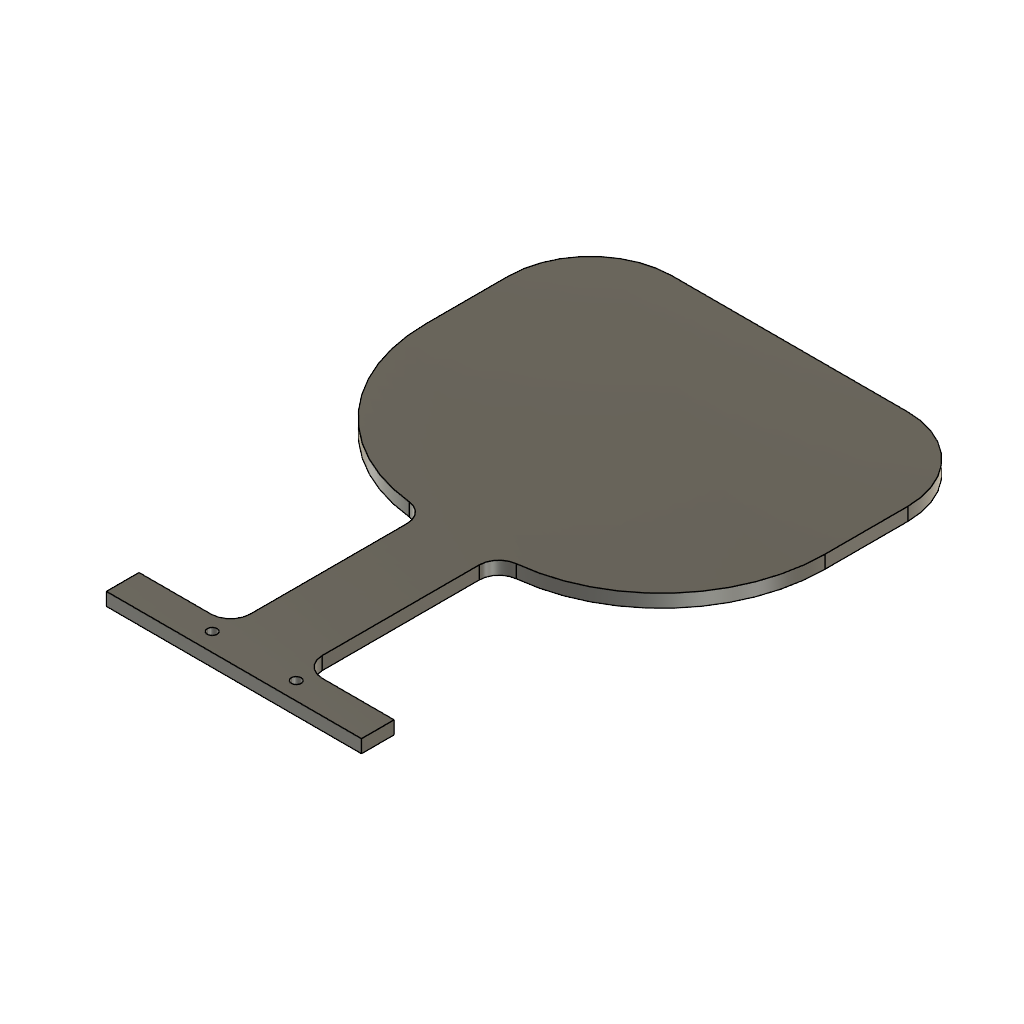
line follower robo chasis (Autodesk Fusion 360 design; units mm, degrees)
part number: 2026-06-19-20-18-20-474
Autodesk Fusion 360 part; units mm, degrees
sketch "Sketch1" plane through (0, 0, 0) normal (0, 0, 1) x (1, 0, 0)
  line L0 (-62, 100) -> (60, 100)
  line L1 (60, 100) -> (60, 0)
  line L2 (60, 0) -> (10, 0)
  line L3 (10, 0) -> (10, -60)
  line L4 (10, -60) -> (38, -60)
  line L5 (38, -60) -> (38, -70)
  line L6 (38, -70) -> (-40, -70)
  line L7 (-40, -70) -> (-40, -60)
  line L8 (-40, -60) -> (-12, -60)
  line L9 (-12, -60) -> (-12, 0)
  line L10 (-12, 0) -> (-62, 0)
  line L11 (-62, 0) -> (-62, 100)
  dimension "d1" = 28
  dimension "d2" = 28
  dimension "d3" = 78
  dimension "d4" = 50
  constraint horizontal L0
  constraint perpendicular L0 L1
  constraint perpendicular L1 L2
  constraint perpendicular L2 L3
  constraint perpendicular L1 L4
  constraint perpendicular L4 L5
  constraint perpendicular L3 L6
  constraint perpendicular L6 L7
  constraint perpendicular L3 L8
  constraint perpendicular L8 L9
  constraint perpendicular L9 L10
  constraint perpendicular L0 L11
  constraint equal L2 L10
  constraint equal L3 L9
  constraint equal L5 L7
  measures "d1" distance of L3.end L4.end
  measures "d2" distance of L7.end L8.end
  measures "d3" distance of L5.end L6.end
  measures "d4" distance of L9.end L10.end
extrude "Extrude1" add sketch "Sketch1" along normal blind 4
fillet "Fillet1" radius 25 2 edges at (60, 100, 2) (-62, 100, 2)
fillet "Fillet2" radius 6 4 edges at (10, 0, 2) (-12, 0, 2) (10, -60, 2) (-12, -60, 2)
hole "Hole1" at (-13.1996, -64.4309, 4) direction (0, 0, -1) diameter 3 depth 10 tip angle 180
hole "Hole2" at (12.6439, -64.5934, 4) direction (0, 0, -1) diameter 3 depth 10 tip angle 180
sketch "Sketch2" plane through (0, 0, 4) normal (0, 0, 1) x (-1, 0, 0)
  circle A0 centre (-12.6439, 64.5934) radius 1.5
  circle A1 centre (13.1996, 64.4309) radius 1.5
  arc A2 (37, -100) -> (62, -75) centre (37, -75) ccw
  line L0 (62, -75) -> (62, 0)
  line L1 (62, 0) -> (18, 0)
  arc A3 (12, 6) -> (18, 0) centre (18, 6) ccw
  line L2 (12, 6) -> (12, 54)
  arc A4 (18, 60) -> (12, 54) centre (18, 54) ccw
  line L3 (18, 60) -> (40, 60)
  line L4 (40, 60) -> (40, 70)
  line L5 (40, 70) -> (-38, 70)
  line L6 (-38, 70) -> (-38, 60)
  line L7 (-38, 60) -> (-16, 60)
  arc A5 (-10, 54) -> (-16, 60) centre (-16, 54) ccw
  line L8 (-10, 54) -> (-10, 6)
  arc A6 (-16, 0) -> (-10, 6) centre (-16, 6) ccw
  line L9 (-16, 0) -> (-60, 0)
  line L10 (-60, 0) -> (-60, -75)
  arc A7 (-60, -75) -> (-35, -100) centre (-35, -75) ccw
  line L11 (-35, -100) -> (37, -100)
  line L12 (62, -70) -> (57, -70)
  line L13 (57, -70) -> (57, -50)
  line L14 (57, -50) -> (62, -50)
  line L15 (62, -50) -> (62, -70)
  line L16 (32, -70) -> (32, -50)
  line L17 (37, -70) -> (32, -70)
  line L18 (37, -50) -> (37, -70)
  line L19 (32, -50) -> (37, -50)
  line L20 (-60, -70) -> (-60, -50)
  line L21 (-55, -70) -> (-60, -70)
  line L22 (-55, -50) -> (-55, -70)
  line L23 (-60, -50) -> (-55, -50)
  line L24 (-35, -70) -> (-35, -50)
  line L25 (-30, -70) -> (-35, -70)
  line L26 (-30, -50) -> (-30, -70)
  line L27 (-35, -50) -> (-30, -50)
  dimension "d17" = 5
  dimension "d18" = 20
  dimension "d19" = 30
  dimension "d20" = 5
  dimension "d21" = 20
  dimension "d22" = 30
  dimension "d23" = 5
  dimension "d24" = 20
  dimension "d25" = 5
  dimension "d26" = 20
  dimension "d27" = 25
  constraint horizontal L12
  constraint vertical L13
  constraint horizontal L14
  constraint vertical L15
  constraint coincident L0 L12.start
  constraint horizontal L17
  constraint vertical L16
  constraint horizontal L19
  constraint vertical L18
  constraint horizontal L25
  constraint vertical L24
  constraint horizontal L27
  constraint vertical L26
  constraint horizontal L21
  constraint vertical L20
  constraint horizontal L23
  constraint vertical L22
  measures "d17" distance of L12.start L12.end
  measures "d18" distance of L12.start L14.end
  measures "d19" distance of L11 L12
  measures "d20" distance of L17.start L16.start
  measures "d21" distance of L17.start L18.start
  measures "d22" distance of L0 L16
  measures "d23" distance of L25.start L24.start
  measures "d24" distance of L25.start L26.start
  measures "d25" distance of L20.start L21.start
  measures "d26" distance of L21.start L22.start
  measures "d27" distance of L10 L24
fillet "Fillet3" radius 50 2 edges at (-62, 0, 2) (60, 0, 2)
extrude "Extrude2" [rolled back] along distance 30 taper angle 0
